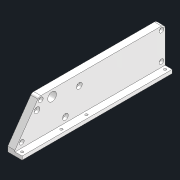
# Autodesk Inventor part: s_base4
Saved by Autodesk Inventor 2022 (Build 260153000, 153)
## iProperties
Created: 2021-08-20
Part Number: s_base4
Material: ABS プラスチック
Document SubType Name: Modeling
Designer: yuta0
Density: 1.06 g/cm^3
Appearance: 滑らか - 白
Mass: 121.862 g
Surface Area: 321.188 cm^2
Volume: 114.964 cm^3
Author: yuta0
Autodesk Inventor part; units mm, degrees
ref_plane "YZ Plane" through (0, 0, 0) normal (1, 0, 0) x (0, 1, 0)
ref_plane "XZ Plane" through (0, 0, 0) normal (0, 1, 0) x (-1, 0, 0)
ref_plane "XY Plane" through (0, 0, 0) normal (0, 0, 1) x (1, 0, 0)
sketch "スケッチ1" plane through (0, 0, 0) normal (0, 0, 1) x (1, 0, 0)
  line L0 (-20, -2.5) -> (20, -2.5)
  line L1 (20, -2.5) -> (20, 2.5)
  line L2 (-20, 2.5) -> (-20, -2.5)
  line L3 (-20, -2.5) -> (20, 2.5) construction
  line L4 (20, -2.5) -> (-20, 2.5) construction
  line L5 (-10, 2.5) -> (10, 2.5)
  line L6 (10, 2.5) -> (10, 52.5)
  line L7 (10, 52.5) -> (-10, 52.5)
  line L8 (-10, 52.5) -> (-10, 2.5)
  line L9 (-10, 2.5) -> (10, 52.5) construction
  line L10 (10, 2.5) -> (-10, 52.5) construction
  line L11 (20, 2.5) -> (10, 2.5)
  line L12 (-10, 2.5) -> (-20, 2.5)
  line L13 (0, 52.5) -> (0, -2.5)
  point P0 (0, 0)
  point P1 (0, 27.5)
  point P2 (0, 27.5)
  point P3 (0, 0)
  dimension "d0" = 20
  dimension "d1" = 50
  dimension "d2" = 5
  dimension "d3" = 10
  constraints: 28 end point, 8 midpoint, 5 parallel, 2 horizontal, 2 perpendicular, 1 vertical alignment
  measures "d0" distance of L6.end L7.end
  measures "d1" distance of L5.end L6.end
  measures "d2" distance of L0.end L1.end
  measures "d3" distance between parallel lines of L8 L2
extrude "押し出し1" add sketch "スケッチ1" along normal mid plane 210 contours L13 L5 L11 L1 L0 | L13 L7 L6 L5
sketch "スケッチ4" plane through (0, -2.5, 105) normal (-1, 0, 0) x (0, 0, 1)
  line L0 (0, 7) -> (-33.61, 55)
  line L1 (-210, 55) -> (0, 55) projected
  line L2 (0, 55) -> (0, 0) projected
  line L3 (0, 5) -> (-210, 5) projected
  point P0 (-105, 2.5)
  dimension "d18" = 35
  dimension "d21" = 2
  constraints: 2 end point, 2 point on line
  measures "d18" angle of L2 L0
  measures "d21" distance from line of L3 L0.start
extrude "押し出し3" cut sketch "スケッチ4" against normal through all
sketch "スケッチ5" plane through (10, 2.5, -105) normal (1, 0, 0) x (0, 0, -1)
  circle A0 centre (-158, 41) radius 6.05
  line L0 (0, 0) -> (-210, 0) projected
  line L1 (-210, 0) -> (-210, 2) projected
  point P0 (-105, -2.5)
  dimension "d22" = 12.1
  dimension "d23" = 41
  dimension "d37" = 52
  constraints: 1 centre point
  measures "d22" diameter of A0
  measures "d23" distance from line of L0 A0.centre
  measures "d37" distance from line of L1 A0.centre
extrude "押し出し4" cut sketch "スケッチ5" against normal blind 10
sketch "スケッチ6" plane through (10, 2.5, 105) normal (0, 1, 0) x (1, 0, 0)
  line L0 (10, 210) -> (10, 0) projected
  line L1 (10, 0) -> (0, 0) projected
  line L2 (0, 210) -> (10, 210) projected
  point P0 (-10, 105)
  point P1 (5, 205)
  point P2 (5, 5)
  point P3 (5, 60)
  point P4 (5, 95)
  dimension "d27" = 5
  dimension "d28" = 5
  dimension "d29" = 5
  dimension "d50" = 35
  dimension "d51" = 55
  constraints: 1 vertical alignment
  measures "d27" distance from line of L0 point (5, 205)
  measures "d28" distance from line of L1 point (5, 5)
  measures "d29" distance from line of L2 point (5, 205)
  measures "d50" distance of point (5, 60) point (5, 95)
  measures "d51" distance of point (5, 5) point (5, 60)
hole "穴2" at (15, 2.5, -100) at (15, 2.5, 100) at (15, 2.5, 45) at (15, 2.5, 10) direction (0, -1, 0) diameter 3.4 end through all clearance for "Socket Head Cap Screw" size "M3" standard "Ansi Metric M Profile"
sketch "スケッチ9" plane through (10, -2.5, -105) normal (-1, 0, 0) x (0, 0, 1)
  circle A0 centre (158, 46) radius 6.05 projected
  line L0 (139.4081, 12.2287) -> (179.2189, 40.1045)
  line L1 (179.2189, 40.1045) -> (159.7173, 67.9557)
  line L2 (159.7173, 67.9557) -> (119.9065, 40.0798)
  line L3 (119.9065, 40.0798) -> (139.4081, 12.2287)
  line L4 (139.4081, 12.2287) -> (159.7173, 67.9557) construction
  line L5 (179.2189, 40.1045) -> (119.9065, 40.0798) construction
  line L6 (210, 7) -> (176.39, 55) projected
  line L7 (158, 46) -> (149.5627, 40.0922) construction
  dimension "d123" = 48.6
  dimension "d124" = 34
  dimension "d125" = 14
  constraints: 14 end point, 4 parallel, 2 midpoint, 1 perpendicular
  measures "d123" distance of L0.start L0.end
  measures "d124" distance of L2.end L0.start
  measures "d125" distance from line of L7.start L1
hole "穴6" at (10, 37.5798, 14.9065) at (10, 9.7287, 34.4081) at (10, 37.6045, 74.2189) direction (-1, 0, 0) diameter 4.5 end through all counterbore diameter 8 counterbore depth 4 clearance for "Socket Head Cap Screw" size "M4" standard "Ansi Metric M Profile"
sketch "スケッチ14" plane through (10, 2.5, -105) normal (1, 0, 0) x (0, 0, -1)
  line L0 (0, 50) -> (0, 0) projected
  line L1 (0, 50) -> (-176.39, 50) projected
  line L2 (0, 0) -> (-210, 0) projected
  line L3 (-176.39, 50) -> (-210, 2) projected
  point P0 (-105, -2.5)
  point P1 (-173.7872, 45)
  point P2 (-200.3951, 7)
  point P3 (-5, 45)
  point P4 (-5, 7)
  dimension "d126" = 5
  dimension "d127" = 5
  dimension "d128" = 7
  dimension "d129" = 5
  dimension "d130" = 5
  constraints: 2 horizontal alignment, 1 vertical alignment
  measures "d126" distance from line of L0 point (-5, 45)
  measures "d127" distance from line of L1 point (-5, 45)
  measures "d128" distance from line of L2 point (-5, 7)
  measures "d129" distance from line of L3 point (-200.395, 7)
  measures "d130" distance from line of L3 point (-173.787, 45)
hole "穴9" at (10, 47.5, 68.7872) at (10, 9.5, 95.3951) at (10, 47.5, -100) at (10, 9.5, -100) direction (-1, 0, 0) diameter 3.4 end through all counterbore diameter 6.5 counterbore depth 4 clearance for "Socket Head Cap Screw" size "M3" standard "Ansi Metric M Profile"
fillet "フィレット1" radius 5 2 edges at (5, 52.5, -105) (5, 52.5, 71.39)
equation "\"d127\" = d126"
equation "\"d129\" = d127"
equation "\"d130\" = d126"
